LinksPassiveAndMotor 8_v2 (Autodesk Fusion 360 design; units mm, degrees)
Autodesk Fusion 360 part; units mm, degrees
sketch "passive link sketch" plane through (0, 0, 0) normal (0, 0, 1) x (1, 0, 0)
  line L0 (-18.5, 6) -> (-18.5, -6) construction
  line L1 (18.5, -6) -> (18.5, 6) construction
  line L2 (18.5, 6) -> (-18.5, -6) construction
  line L3 (-18.5, 6) -> (18.5, -6) construction
  circle A0 centre (12.5, 0) radius 1
  circle A1 centre (12.5, 0) radius 2.975
  circle A2 centre (12.5, 0) radius 6
  line L4 (0, 6) -> (0, -15) construction
  line L5 (12.5, 6) -> (0, 6)
  line L6 (0, -6) -> (12.5, -6)
  line L7 (12.5, -6) -> (12.5, 6)
  line L8 (12.5, 6) -> (-12.5, -6) construction
  line L9 (-12.5, 6) -> (12.5, -6) construction
  line L10 (18.5, 6) -> (0, 6) construction
  line L11 (-12.5, 6) -> (-18.5, 6) construction
  line L12 (-18.5, -6) -> (-12.5, -6) construction
  line L13 (0, -6) -> (18.5, -6) construction
  line L14 (0, -6) -> (-18.5, -6) construction
  line L15 (-12.5, -6) -> (-12.5, 6)
  line L16 (-18.5, 6) -> (0, 6) construction
  circle A3 centre (-12.5, 0) radius 6
  circle A4 centre (-12.5, 0) radius 2.975
  circle A5 centre (-12.5, 0) radius 1
  line L17 (0, -6) -> (-12.5, -6)
  line L18 (-12.5, 6) -> (0, 6)
  dimension "d2" = 12
  dimension "d3" = 2
  dimension "d4" = 5.95
  dimension "d5" = 12
  dimension "d6" = 12.5
  dimension "d7" = 25
  constraint horizontal L10
  constraint perpendicular L0 L10
  constraint parallel L10 L12
  constraint parallel L0 L1
  constraint coincident L2 origin
  constraint coincident L3 origin
  constraint concentric A0 A1
  constraint concentric A0 A2
  constraint perpendicular L4 L12
  constraint horizontal origin A0.centre
  constraint horizontal L5
  constraint parallel L5 L6
  constraint coincident A2 L5.start
  constraint coincident L8 origin
  constraint coincident L9 origin
  constraint collinear L10 L11
  constraint coincident L4 L6.start
  constraint collinear L12 L13
  constraint symmetric L1.end L4 L0.start
  constraint symmetric L1.start L4 L0.end
  constraint symmetric A0 L4 A5
  constraint symmetric A1 L4 A4
  constraint symmetric A2 L4 A3
  constraint symmetric L4 L5.start L9.start
  constraint symmetric L4 L6.end L8.end
  constraint symmetric L4 L5.end L10.end
  constraint symmetric L4 L6.start L13.start
  constraint perpendicular L15 L18
  measures "d2" distance of L0.start L0.end
  measures "d3" diameter of A0
  measures "d4" diameter of A1
  measures "d5" diameter of A2
  measures "d6" distance of origin A0.centre
  measures "d7" distance of L8.end L6.end
extrude "base" add sketch "passive link sketch" along normal mid plane 10 contours A0 L7 | A0 A1 L7 | A1 A2 L7 | A2 L5 L6 A3 L17 L18 | L15 A3 A4 | L15 A4 A5 | L15 A5 picked at (12.1897, -0.1218) picked at (11.3665, -2.0131) picked at (9.947, 4.2738) picked at (-7.5388, -0.4258) picked at (-10.1968, -0.1886) picked at (-12.0298, -0.2997) makes body 1
extrude "l  big cyl" add sketch "passive link sketch" along normal blind -7 and the other way blind -5 contours L15 A3 A4 | L15 A3 A4 | L15 A4 A5 | L15 A4 A5 bodies 1
extrude "Extrude7" add sketch "passive link sketch" against normal blind 12 contours L15 A4 A5 | L15 A4 A5 bodies 1
fillet "Fillet4" radius 0.3 1 edges at (-15.2737, 1.0758, -12) on bodies 1
extrude "Extrude8" cut sketch "passive link sketch" along normal blind 5 and the other way blind 12 contours L15 A5 | L15 A5 bodies 1
extrude "r big cyl" add sketch "passive link sketch" along normal blind 7 and the other way blind 5 contours A0 A1 L7 | A0 A1 L7 | A1 A2 L7 | A1 A2 L7 bodies 1
extrude "r small cyl" add sketch "passive link sketch" along normal blind 12 and the other way blind 5 contours A0 A1 L7 | A0 A1 L7 bodies 1
extrude "Extrude9" cut sketch "passive link sketch" along normal blind 12 and the other way blind 5 contours A0 L7 | A0 L7 bodies 1
fillet "Fillet1" radius 0.3 1 edges at (9.7263, -1.0758, 12) on bodies 1
sketch "top nut" plane through (0, 0, 5) normal (0, 0, 1) x (-1, 0, 0)
  line L0 (12.5, 6) -> (-12.5, 6)
  arc A0 (-12.5, -6) -> (-12.5, 6) centre (-12.5, 0) ccw
  line L1 (-12.5, -6) -> (12.5, -6)
  circle A1 centre (12.5, 0) radius 2.5 construction
  line L2 (14.5842, -1.3806) -> (14.7377, 1.1147)
  line L3 (14.7377, 1.1147) -> (12.6535, 2.4953)
  line L4 (12.6535, 2.4953) -> (10.4158, 1.3806)
  line L5 (10.4158, 1.3806) -> (10.2623, -1.1147)
  line L6 (10.2623, -1.1147) -> (12.3465, -2.4953)
  line L7 (12.3465, -2.4953) -> (14.5842, -1.3806)
  circle A2 centre (12.5, 0) radius 1
  arc A3 (12.5, -6) -> (12.5, 6) centre (12.5, 0) ccw
  point P0 (12.5, 0)
  dimension "d35" = 5
  constraint coincident P0 A1.centre
  constraint coincident A1 L2.start
  measures "d35" diameter of A1
extrude "Extrude10" cut sketch "top nut" against normal blind 4 contours L2 L3 L4 L5 L6 L7 bodies 1
sketch "bottom nut" plane through (0, 0, -5) normal (0, 0, -1) x (1, 0, 0)
  circle A0 centre (12.5, 0) radius 2.5 construction
  arc A1 (-12.5, -6) -> (-12.5, 6) centre (-12.5, 0) ccw
  line L0 (-12.5, -6) -> (12.5, -6)
  line L1 (12.5, 6) -> (-12.5, 6)
  circle A2 centre (12.5, 0) radius 1
  arc A3 (12.5, -6) -> (12.5, 6) centre (12.5, 0) ccw
  line L2 (12.5, -2.5) -> (14.6651, -1.25)
  line L3 (14.6651, -1.25) -> (14.6651, 1.25)
  line L4 (14.6651, 1.25) -> (12.5, 2.5)
  line L5 (12.5, 2.5) -> (10.3349, 1.25)
  line L6 (10.3349, 1.25) -> (10.3349, -1.25)
  line L7 (10.3349, -1.25) -> (12.5, -2.5)
  point P0 (12.5, 0)
  point P1 (12.5, 0)
  dimension "d38" = 5
  constraint coincident P0 A0.centre
  constraint coincident P1 P0
  constraint coincident A0 L2.start
  measures "d38" diameter of A0
extrude "Extrude11" cut sketch "bottom nut" against normal blind 4 contours A2 | L2 L3 L4 L5 L6 L7 bodies 1
sketch "motorLinkSketch" plane through (0, 0, 0) normal (0, 0, 1) x (1, 0, 0) in component "MotorLinkComponent"
  circle A0 centre (-12.5, 0) radius 1
  line L0 (18.5, 6) -> (-18.5, -6) construction
  circle A1 centre (-12.5, 0) radius 2.975
  line L1 (-12.5, 6) -> (-18.5, 6) construction
  line L2 (-18.5, -6) -> (-12.5, -6) construction
  circle A2 centre (12.5, 0) radius 1
  line L3 (0, -6) -> (-12.5, -6)
  line L4 (-12.5, -6) -> (-12.5, 6)
  line L5 (-12.5, 6) -> (0, 6)
  line L6 (14.65, -1.462) -> (14.65, 1.462)
  line L7 (12.5, 6) -> (0, 6)
  line L8 (18.5, 6) -> (0, 6) construction
  line L9 (0, -6) -> (12.5, -6)
  line L10 (-18.5, 6) -> (-18.5, -6) construction
  line L11 (0, 6) -> (0, -15) construction
  line L12 (18.5, -6) -> (18.5, 6) construction
  line L13 (-18.5, 6) -> (0, 6) construction
  line L14 (0, -6) -> (18.5, -6) construction
  circle A3 centre (12.5, 0) radius 2.6
  circle A4 centre (-12.5, 0) radius 6
  line L15 (0, -6) -> (-18.5, -6) construction
  line L16 (-18.5, 6) -> (18.5, -6) construction
  line L17 (12.5, 6) -> (-12.5, -6) construction
  line L18 (12.5, -6) -> (12.5, 6)
  circle A5 centre (12.5, 0) radius 6
  line L19 (-12.5, 6) -> (12.5, -6) construction
  dimension "d65" = 12
  dimension "d66" = 2
  dimension "d67" = 5.2
  dimension "d68" = 12
  dimension "d69" = 12.5
  dimension "d70" = 25
  dimension "d71" = 2.15
  dimension "d72" = 5.95
  constraint horizontal L8
  constraint perpendicular L8 L10
  constraint parallel L2 L8
  constraint parallel L10 L12
  constraint coincident origin L0
  constraint coincident origin L16
  constraint concentric A2 A3
  constraint concentric A2 A5
  constraint perpendicular L2 L11
  constraint horizontal A2.centre origin
  constraint horizontal L7
  constraint parallel L7 L9
  constraint coincident L7.start A5
  constraint coincident origin L17
  constraint coincident origin L19
  constraint collinear L1 L8
  constraint coincident L3.start L11
  constraint collinear L2 L14
  constraint symmetric L1.end L0.start L11
  constraint symmetric L0.end L12.start L11
  constraint symmetric A0 A2 L11
  constraint symmetric L11 A4 A5
  constraint symmetric L7.start L1.start L11
  constraint symmetric L9.end L2.end L11
  constraint symmetric L5.end L7.end L11
  constraint symmetric L3.start L9.start L11
  constraint perpendicular L4 L5
  constraint coincident L6.start A3
  constraint coincident L6.end A3
  constraint vertical L6
  measures "d65" distance of L1.end L0.end
  measures "d66" diameter of A2
  measures "d67" diameter of A3
  measures "d68" diameter of A5
  measures "d69" distance of A2.centre origin
  measures "d70" distance of L9.end L2.end
  measures "d71" distance of A2.centre L6
  measures "d72" diameter of A1
extrude "Extrude5" add sketch "motorLinkSketch" along normal blind 5 and the other way blind 5 separate body contours A0 L4 | A0 A1 L4 | A1 L4 A4 | L3 L5 L7 L9 A4 A5 | A3 L18 A5 | A2 A3 L18 | A2 L18 picked at (-12.2249, 0.2804) picked at (-10.1968, -0.1886) picked at (-7.5388, -0.4258) picked at (10.0174, 4.1705) picked at (12.1897, -0.1218) makes body 2 in component "MotorLinkComponent"
extrude "Extrude3" add sketch "motorLinkSketch" along normal blind 5 and the other way blind 7 separate body contours A0 A1 L4 | A0 A1 L4 | A1 L4 A4 | A1 L4 A4 makes body 3 in component "MotorLinkComponent"
extrude "Extrude4" add sketch "motorLinkSketch" along normal blind 5 and the other way blind 12 separate body contours A0 A1 L4 | A0 A1 L4 makes body 4 in component "MotorLinkComponent"
extrude "Extrude12" [suppressed]
extrude "Extrude7'" cut sketch "motorLinkSketch" along normal blind 5 and the other way blind 12 contours A0 L4 | A0 L4 bodies 2 in component "MotorLinkComponent"
fillet "Fillet1'" radius 0.3 1 edges at (-15.2737, 1.0758, -12) on bodies 4 in component "MotorLinkComponent"
extrude "Extrude2" add sketch "motorLinkSketch" along normal blind 10.9 and the other way blind 5 separate body contours A3 L18 A5 | A3 L18 A5 | A2 A3 L18 | A2 L6 A3 L18 | L6 A3 makes body 5 in component "MotorLinkComponent"
extrude "Extrude1" cut sketch "motorLinkSketch" along normal blind 10.9 and the other way blind 5 contours A2 A3 L18 | A2 L6 A3 L18 | A2 L18 | A2 L18 bodies 5 in component "MotorLinkComponent"
fillet "Fillet2" radius 1 1 edges at (6.906, -2.1697, 10.9) on bodies 5 in component "MotorLinkComponent"
sketch "top nut (2)" plane through (0, 0, 5) normal (0, 0, 1) x (-1, 0, 0) in component "MotorLinkComponent"
  circle A0 centre (12.5, 0) radius 1
  circle A1 centre (12.5, 0) radius 2.975
  line L0 (14.5842, -1.3806) -> (14.7377, 1.1147)
  line L1 (12.3465, -2.4953) -> (14.5842, -1.3806)
  line L2 (10.2623, -1.1147) -> (12.3465, -2.4953)
  circle A2 centre (12.5, 0) radius 1
  circle A3 centre (12.5, 0) radius 2.5 construction
  line L3 (12.6535, 2.4953) -> (10.4158, 1.3806)
  arc A4 (12.5, -6) -> (12.5, 6) centre (12.5, 0) ccw
  line L4 (10.4158, 1.3806) -> (10.2623, -1.1147)
  line L5 (14.7377, 1.1147) -> (12.6535, 2.4953)
  point P0 (12.5, 0)
  dimension "d106" = 5
  constraint coincident P0 A0.centre
  constraint coincident L0.start A3
  measures "d106" diameter of A3
extrude "Extrude6" cut sketch "top nut (2)" against normal blind 4 contours L0 L1 L2 L3 L4 L5 bodies 2 3 4 in component "MotorLinkComponent"
sketch "spacer" plane through (0, 0, 0) normal (0, 0, 1) x (1, 0, 0)
  circle A0 centre (-61, 0) radius 4
  circle A1 centre (-61, 0) radius 1
  dimension "d123" = 8
  dimension "d126" = 2
  constraint concentric A0 A1
  measures "d123" diameter of A0
  measures "d126" diameter of A1
extrude "Extrude16" add sketch "spacer" along normal blind 3 separate body makes body 6
hole "Hole1" at (18.5, 0, 7.6715) direction (-1, 0, 0) diameter 2 depth 5 tip angle 118 bodies 5 in component "MotorLinkComponent"
component "MotorLinkComponent" placed x (1, 0, 0) y (0, 1, 0) z (0, 0, 1) at (40, 0, 0)
equation "d2 = BigBarrelDiam"
equation "d3 = smallerHoleDiam"
equation "d4 = nipDiameter"
equation "d5 = BigBarrelDiam"
equation "d8 = rect / 2"
equation "d10 = rect / 2 + shoulder"
equation "d12 = rect / 2 + shoulder + regularNip"
equation "d16 = -rect / 2 - shoulder"
equation "d20 = -rect / 2 - shoulder - regularNip"
equation "d22 = rect / 2"
equation "d24 = rect + shoulder"
equation "d25 = 0.0 °"
equation "d26 = rect / 2 + shoulder + regularNip"
equation "d36 = -hex"
equation "d39 = -hex"
equation "d48 = rect / 2"
equation "d49 = 0.0 °"
equation "d50 = rect / 2"
equation "d51 = 0.0 °"
equation "d52 = -rect / 2"
equation "d53 = 0.0 °"
equation "d54 = rect / 2"
equation "d55 = 0.0 °"
equation "rect = 10 mm"
equation "shoulder = 2 mm"
equation "regularNip = 5 mm"
equation "hex = 4 mm"
equation "nipDiameter = 5.95 mm"
equation "BigBarrelDiam = 12 mm"
equation "smallerHoleDiam = 2 mm"
equation "d66 = smallerHoleDiam"
equation "d67 = motorShaftDiameter"
equation "d68 = BigBarrelDiam"
equation "d72 = nipDiameter"
equation "motorShaftDiameter = 5.2 mm"
equation "d76 = rect / 2"
equation "d80 = rect / 2 + shaftNip"
equation "d82 = rect / 2"
equation "d83 = 0.0 °"
equation "d84 = rect / 2 + shaftNip"
equation "d86 = rect / 2"
equation "d87 = 0.0 °"
equation "d88 = rect / 2"
equation "d90 = rect / 2 + shoulder"
equation "d91 = 0.0 °"
equation "d92 = rect / 2"
equation "d94 = rect / 2 + shoulder + regularNip"
equation "d95 = 0.0 °"
equation "shaftNip = 5.9 mm"
equation "rectLen = 25 mm"
equation "d98 = rect / 2"
equation "d100 = rect / 2"
equation "d101 = 0.0 °"
equation "d109 = rect / 2"
equation "d111 = rect / 2 + shoulder + regularNip"
equation "d112 = 0.0 °"
equation "d113 = rect / 2 + shoulder + regularNip"
equation "d114 = 0.0 °"
named bodies: "PassiveLinkBody", "big barrel motor shaft", "big barrel", "nip", "rect", "spacer"
